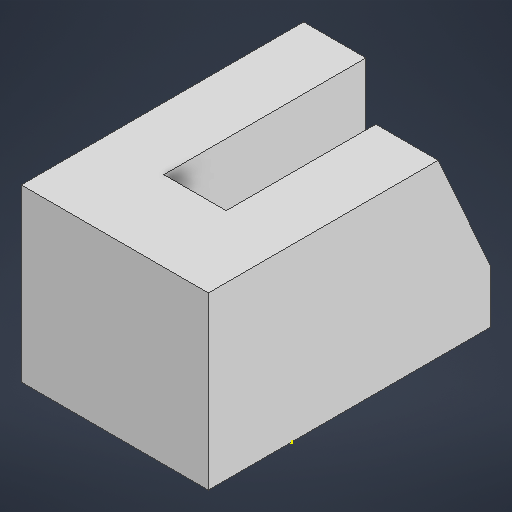
# Autodesk Inventor part: trabalho well1
Saved by Autodesk Inventor 2025.1 (Build 291241000, 241)
## iProperties
Created: 2024-08-15
Part Number: trabalho well1
Material: Generic
Document SubType Name: Modeling
Designer: PC-EDUCERE
Density: 1 g/cm^3
Appearance: Default
Author: PC-EDUCERE
Autodesk Inventor part; units mm, degrees
ref_plane "YZ Plane" through (0, 0, 0) normal (1, 0, 0) x (0, 1, 0)
ref_plane "XZ Plane" through (0, 0, 0) normal (0, 1, 0) x (-1, 0, 0)
ref_plane "XY Plane" through (0, 0, 0) normal (0, 0, 1) x (1, 0, 0)
sketch "Sketch1" plane through (0, 0, 0) normal (0, 1, 0) x (-1, 0, 0)
  line L0 (23.5896, 25.2844) -> (-33.4104, 25.2844)
  line L1 (-33.4104, 25.2844) -> (-33.4104, -60.7156)
  line L2 (-33.4104, -60.7156) -> (-14.4104, -60.7156)
  line L3 (-14.4104, -60.7156) -> (-14.4104, 0.867)
  line L4 (-14.4104, 0.867) -> (4.5896, 0.867)
  line L5 (4.5896, 0.867) -> (4.5896, -60.7156)
  line L6 (4.5896, -60.7156) -> (23.5896, -60.7156)
  line L7 (23.5896, -60.7156) -> (23.5896, 25.2844)
  point P0 (0, 0)
  dimension "d0" = 19
  dimension "d1" = 19
  dimension "d2" = 19
  dimension "d3" = 86
  dimension "d9" = 57
  dimension "d10" = 86
  constraints: 16 end point, 4 perpendicular, 2 horizontal, 1 vertical
  measures "d0" distance of L5.end L6.end
  measures "d1" distance of L1.end L2.end
  measures "d2" distance of L3.end L4.end
  measures "d3" distance of L0.end L1.end
  measures "d9" distance of L0.start L0.end
  measures "d10" distance of L6.end L0.start
extrude "Extrusion1" add sketch "Sketch1" along normal blind 52
sketch "Sketch2" plane through (33.4104, 0, -60.7156) normal (1, 0, 0) x (0, 0, -1)
  line L0 (0, 52) -> (-61.5826, 52) projected
  line L1 (0, 0) -> (0, 52) projected
  line L2 (0, 10.9784) -> (0, 52)
  line L3 (0, 0) -> (0, 52) projected
  line L4 (0, 10.9784) -> (0, 52)
  line L5 (0, 52) -> (-1.0633, 52)
  line L6 (0, 52) -> (-86, 52) projected
  line L7 (0, 52) -> (-14.1637, 52)
  line L8 (0, 10.9784) -> (0, 52)
  line L9 (-86, 52) -> (0, 52)
  line L10 (0, 52) -> (0, 0)
  line L11 (0, 0) -> (-86, 0)
  line L12 (-86, 0) -> (-86, 52)
  line L13 (0, 0) -> (0, 16)
  line L14 (-86, 52) -> (-16, 52)
  line L15 (-16, 52) -> (0, 16)
  point P0 (-60.7156, 0)
  point P1 (0, 52)
  dimension "d11" = 16
  dimension "d12" = 70
  constraints: 24 end point, 5 point on line, 2 collinear, 2 parallel, 1 horizontal, 1 perpendicular
  measures "d11" distance of L3.start L13.end
  measures "d12" distance of L6.end L14.end
sketch "Sketch3" plane through (33.4104, 0, -60.7156) normal (1, 0, 0) x (0, 0, -1)
  point P0 (-60.7156, 0)
extrude "Extrusion2" cut sketch "Sketch2" against normal blind 19.3 contours L1 L15 L0
body "Solid1"
